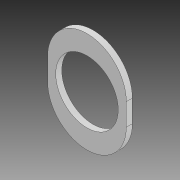
# Autodesk Inventor part: housingPlate
Saved by Autodesk Inventor 2020 (Build 240168000, 168)
## iProperties
Created: 2020-11-25
Part Number: housingPlate
Material: Generic
Document SubType Name: Modeling
Designer: DDeGo
Density: 1 g/cm^3
Appearance: Default
Author: DDeGo
Autodesk Inventor part; units mm, degrees
ref_plane "YZ Plane" through (0, 0, 0) normal (1, 0, 0) x (0, 1, 0)
ref_plane "XZ Plane" through (0, 0, 0) normal (0, 1, 0) x (-1, 0, 0)
ref_plane "XY Plane" through (0, 0, 0) normal (0, 0, 1) x (1, 0, 0)
sketch "Sketch1" plane through (0, 0, 0) normal (0, 0, 1) x (1, 0, 0)
  line L0 (0, 0) -> (0, 5.5) construction
  arc A0 (16.4602, 1.25) -> (-16.4602, 1.25) centre (0, 5.5) ccw construction
  line L1 (0, 0) -> (0, -5.5) construction
  arc A1 (-16.4602, -1.25) -> (16.4602, -1.25) centre (0, -5.5) ccw construction
  line L2 (0, 5.5) -> (0, -5.5) construction
  line L3 (-19.5, 5.5) -> (-19.5, -5.5)
  line L4 (19.5, -5.5) -> (19.5, 5.5)
  arc A2 (19.5, 5.5) -> (-19.5, 5.5) centre (0, 5.5) ccw
  arc A3 (-19.5, -5.5) -> (19.5, -5.5) centre (0, -5.5) ccw
  arc A4 (-16.4602, -1.25) -> (-16.4602, 1.25) centre (-21.3014, 0) ccw construction
  arc A5 (16.4602, 1.25) -> (16.4602, -1.25) centre (21.3014, 0) ccw construction
  line L5 (0, 5.5) -> (0, -5.5) construction
  circle A6 centre (0, 0) radius 15.5
  dimension "d0" = 11
  dimension "d1" = 17
  dimension "d2" = 2.5
  dimension "d3" = 5
  dimension "d4" = 39
  dimension "d8" = 31
  constraints: 16 end point, 12 point on circle, 8 tangent, 7 centre point, 4 coincident, 3 vertical, 2 collinear, 2 equal radius, 2 midpoint, 1 parallel
  measures "d0" distance of L1.end L0.end
  measures "d1" radius of A0
  measures "d2" radial gap between concentric circles of A3 A1
  measures "d3" radius of A4
  measures "d4" distance between parallel lines of L4 L3
  measures "d8" diameter of A6
extrude "Extrusion1" add sketch "Sketch1" along normal blind 3
body "Solid1"
